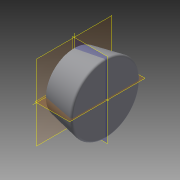
# Autodesk Inventor part: ScheinwerferFront
Saved by Autodesk Inventor 2015 (Build 190159000, 159)
## iProperties
Created: 2019-02-15
Part Number: ScheinwerferFront
Material: Generisch
Document SubType Name: Modeling
Designer: Boris
Density: 1 g/cm^3
Appearance: Vorgabe
Author: Boris
Autodesk Inventor part; units mm, degrees
sketch "Skizze1" plane through (0, 0, 0) normal (0, 0, 1) x (1, 0, 0)
  line L0 (4, 3.3) -> (0, 2.5)
  line L1 (4.5, 4.9297) -> (0, 4.0297)
  line L2 (0, 2.5) -> (0, 4.0297)
  line L3 (4.5, 4.9297) -> (4.5, 3.4)
  line L4 (-0.9, 0) -> (5.4, 0) projected
  line L5 (4.5, 3.4) -> (4.5, 0)
  line L6 (4, 3.3) -> (4, 0)
  line L7 (4, 0) -> (4.5, 0)
  point P0 (0, 0)
  dimension "d53" = 2.5
  dimension "d55" = 1.5
  dimension "d61" = 4.5
  dimension "d62" = 0.5
  constraints: 14 end point, 2 parallel, 2 vertical, 1 collinear, 1 perpendicular, 1 point on line
  measures "d53" distance of point (0, 0) L0.end
  measures "d55" distance between parallel lines of L0 L1
  measures "d61" distance between parallel lines of L3 L2
  measures "d62" distance between parallel lines of L5 L6
revolve "Umdrehung1" add sketch "Skizze1" angle 360 about axis through (-10, 0, 0) along (1, 0, 0)
fillet "Rundung8" radius 1.5 1 edges at (0, -2.5, 0)
fillet "Rundung9" radius 0.25 1 edges at (4.5, -4.9297, 0)
